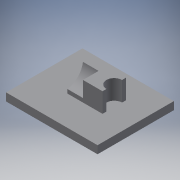
# Autodesk Inventor part: isosketch4.0001
Saved by Autodesk Inventor 2016 (Build 200138000, 138)
## iProperties
Created: 2005-07-26
Part Number: isosketch4.0001
Document SubType Name: Modeling
Designer: waunakee
Material: Generic
Density: 1 g/cm^3
Appearance: Default
Author: waunakee
Autodesk Inventor part; units mm, degrees
ref_plane "YZ Plane" through (0, 0, 0) normal (1, 0, 0) x (0, 1, 0)
ref_plane "XZ Plane" through (0, 0, 0) normal (0, 1, 0) x (-1, 0, 0)
ref_plane "XY Plane" through (0, 0, 0) normal (0, 0, 1) x (1, 0, 0)
sketch "Sketch1" plane through (0, 0, 0) normal (0, 0, 1) x (1, 0, 0)
  line L0 (-36.0465, 32.6227) -> (21.1035, 32.6227)
  line L1 (21.1035, 32.6227) -> (21.1035, 0.8727)
  line L2 (21.1035, 0.8727) -> (-36.0465, 0.8727)
  line L3 (-36.0465, 0.8727) -> (-36.0465, 32.6227)
  dimension "d0" = 57.15
  dimension "d1" = 31.75
  constraints: 8 end point, 2 parallel, 1 horizontal, 1 perpendicular
  measures "d0" distance of L0.start L0.end
  measures "d1" distance of L2.end L0.start
extrude "Extrusion1" add sketch "Sketch1" against normal blind 38.1
sketch "Sketch2" plane through (-36.0465, 32.6227, 0) normal (0, 1, 0) x (1, 0, 0)
  line L0 (57.15, 0) -> (57.15, 38.1) projected
  arc A0 (57.15, 31.75) -> (57.15, 6.35) centre (57.15, 19.05) ccw
  dimension "d4" = 25.4
  constraints: 2 point on circle, 2 point on line, 1 centre point, 1 midpoint
  measures "d4" diameter of A0
extrude "Extrusion2" cut sketch "Sketch2" against normal through all
sketch "Sketch3" plane through (-36.0465, 0.8727, 0) normal (-1, 0, 0) x (0, 0, 1)
  line L0 (0, 0) -> (0, 31.75) projected
  line L1 (0, 31.75) -> (-38.1, 31.75) projected
  arc A0 (-25.4, 31.75) -> (0, 6.35) centre (3.8431, 35.5931) ccw
  dimension "d7" = 12.7
  dimension "d8" = 6.35
  constraints: 2 point on circle, 2 point on line, 1 centre point
  measures "d7" distance of L1.end A0.start
  measures "d8" distance of L0.start A0.end
extrude "Extrusion3" cut sketch "Sketch3" against normal blind 25.4
sketch "Sketch4" plane through (-36.0465, 0.8727, 0) normal (0, -1, 0) x (1, 0, 0)
  line L0 (-51.1761, 48.15) -> (97.2207, 48.15)
  line L1 (97.2207, 48.15) -> (97.2207, -75.7771)
  line L2 (97.2207, -75.7771) -> (-51.1761, -75.7771)
  line L3 (-51.1761, -75.7771) -> (-51.1761, 48.15)
  point P0 (36.0465, 0)
  constraints: 8 end point, 2 parallel, 1 horizontal, 1 perpendicular
extrude "Extrusion4" add sketch "Sketch4" along normal blind 12.7
body "Solid1"
